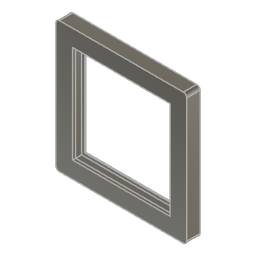
wand handle (Autodesk Fusion 360 archive; units mm, degrees)
design "noita spell v2"
Autodesk Fusion 360 part; units mm, degrees
sketch "Sketch1" plane through (0, 0, 0) normal (0, 1, 0) x (1, 0, 0)
  line L0 (0, 0) -> (38.1, 0)
  line L1 (38.1, 0) -> (38.1, -38.1)
  line L2 (38.1, -38.1) -> (0, -38.1)
  line L3 (0, -38.1) -> (0, 0)
  circle A0 centre (19.05, -40.55) radius 1.25
  line L4 (-4.9, -39.3) -> (43, -39.3) construction
  line L5 (-4.9, -41.8) -> (43, -41.8) construction
  line L6 (0, -19.05) -> (38.1, -19.05)
  line L7 (19.05, 0) -> (19.05, -38.1)
  line L8 (-3.65, 4.9) -> (41.75, 4.9)
  line L9 (43, 3.65) -> (43, -41.75)
  line L10 (41.75, -43) -> (-3.65, -43)
  line L11 (-4.9, -41.75) -> (-4.9, 3.65)
  circle A1 centre (-2.45, -40.55) radius 1.25
  line L12 (-3.7, -43) -> (-3.7, 4.9) construction
  line L13 (-1.2, -43) -> (-1.2, 4.9) construction
  line L14 (39.3, -43) -> (39.3, 4.9) construction
  line L15 (41.8, 4.9) -> (41.8, -43) construction
  line L16 (-4.9, 3.7) -> (43, 3.7) construction
  line L17 (43, 1.2) -> (-4.9, 1.2) construction
  circle A2 centre (40.55, -40.55) radius 1.25
  circle A3 centre (40.55, -19.05) radius 1.25
  circle A4 centre (40.55, 2.45) radius 1.25
  circle A5 centre (19.05, 2.45) radius 1.25
  circle A6 centre (-2.45, 2.45) radius 1.25
  circle A7 centre (-2.45, -19.05) radius 1.25
  arc A8 (-4.9, -41.75) -> (-3.65, -43) centre (-3.65, -41.75) ccw
  arc A9 (41.75, -43) -> (43, -41.75) centre (41.75, -41.75) ccw
  arc A10 (43, 3.65) -> (41.75, 4.9) centre (41.75, 3.65) ccw
  arc A11 (-3.65, 4.9) -> (-4.9, 3.65) centre (-3.65, 3.65) ccw
  line L18 (1.2, -36.9) -> (36.9, -36.9)
  line L19 (36.9, -36.9) -> (36.9, -1.2)
  line L20 (36.9, -1.2) -> (1.2, -1.2)
  line L21 (1.2, -1.2) -> (1.2, -36.9)
  dimension "d1" = 38.1
  dimension "d2" = 38.1
  dimension "d3" = 2.5
  dimension "d4" = 1.2
  dimension "d5" = 1.2
  dimension "d8" = 2.5
  dimension "d9" = 1.2
  dimension "d10" = 1.2
  dimension "d11" = 1.2
  dimension "d13" = 1.2
  dimension "d14" = 1.2
  dimension "d15" = 1.2
  dimension "d16" = 2.5
  dimension "d17" = 1.25
  dimension "d18" = 1.2
  dimension "d19" = 1.2
  dimension "d20" = 1.2
  dimension "d21" = 1.2
  constraint horizontal L0
  constraint vertical L1
  constraint horizontal L2
  constraint vertical L3
  constraint coincident L0.start L3.end
  constraint horizontal L4
  constraint tangent A0 L4
  constraint horizontal L5
  constraint tangent A0 L5
  constraint midpoint L3 L6.start
  constraint midpoint L1 L6.end
  constraint midpoint L0 L7.start
  constraint midpoint L2 L7.end
  constraint horizontal L8
  constraint vertical L9
  constraint horizontal L10
  constraint vertical L11
  constraint coincident L4.start L11
  constraint coincident L4.end L9
  constraint coincident L5.end L9
  constraint coincident L5.start L11
  constraint coincident A0.centre L7
  constraint coincident L10 L12.start
  constraint coincident L8 L12.end
  constraint perpendicular L8 L12
  constraint tangent A1 L12
  constraint coincident L10 L13.start
  constraint coincident L8 L13.end
  constraint perpendicular L8 L13
  constraint tangent A1 L13
  constraint coincident L10 L14.start
  constraint coincident L8 L14.end
  constraint perpendicular L8 L14
  constraint coincident L8 L15.start
  constraint coincident L10 L15.end
  constraint perpendicular L10 L15
  constraint coincident L11 L16.start
  constraint coincident L9 L16.end
  constraint perpendicular L9 L16
  constraint coincident L9 L17.start
  constraint coincident L11 L17.end
  constraint perpendicular L11 L17
  constraint tangent L4 A2
  constraint tangent L15 A2
  constraint tangent L14 A2
  constraint tangent L15 A3
  constraint tangent L16 A4
  constraint tangent L16 A5
  constraint tangent L12 A6
  constraint tangent L17 A6
  constraint tangent L16 A6
  constraint tangent L14 A4
  constraint tangent L15 A4
  constraint tangent L17 A5
  constraint tangent L17 A4
  constraint tangent L12 A7
  constraint tangent L13 A7
  constraint tangent L14 A3
  constraint coincident L6 A3.centre
  constraint coincident L6 A7.centre
  constraint coincident L7 A5.centre
  constraint tangent L5 A1
  constraint tangent L10 A8
  constraint tangent L11 A8
  constraint tangent L9 A9
  constraint tangent L10 A9
  constraint equal A8 A9
  constraint tangent L8 A10
  constraint tangent L9 A10
  constraint equal A8 A10
  constraint tangent L8 A11
  constraint tangent L11 A11
  constraint equal A8 A11
  constraint horizontal L18
  constraint vertical L19
  constraint horizontal L20
  constraint vertical L21
  measures "d1" distance of L1.end L2.end
  measures "d2" distance of L0.start L2.end
  measures "d3" diameter of A0
  measures "d4" distance of L2 L4
  measures "d5" distance of L5 L10
  measures "d8" diameter of A1
  measures "d9" distance of L11 L12
  measures "d10" distance of L3 L13
  measures "d11" distance of L1 L14
  measures "d13" distance of L9 L15
  measures "d14" distance of L8 L16
  measures "d15" distance of L0 L17
  measures "d16" diameter of A2
  measures "d17" radius of A8
  measures "d18" distance of L2 L18
  measures "d19" distance of L3 L21
  measures "d20" distance of L0 L20
  measures "d21" distance of L1 L19
extrude "Extrude1" add sketch "Sketch1" along normal blind 0.4 contours L0 L3 L6 L7 L20 L21 | L0 L1 L6 L7 L19 L20 | L2 L3 L6 L7 L18 L21 | L1 L2 L6 L7 L18 L19 | A0 | L8 L9 L10 L11 A8 A9 A10 A11 | A1 | A2 | A3 | A4 | A5 | A6 | A7
extrude "Extrude2" add sketch "Sketch1" against normal blind 4.1
ref_plane "WorkPlane1" through (19.05, -3.3782, 19.05) normal (0, -1, 0) x (-1, 0, 0)
sketch "Sketch2" plane through (0, -3.3782, 0) normal (0, -1, 0) x (-1, 0, 0)
  line L0 (-1.2, -1.2) -> (-1.2, -36.9)
  line L1 (-1.2, -36.9) -> (-36.9, -36.9)
  line L2 (-36.9, -36.9) -> (-36.9, -1.2)
  line L3 (-36.9, -1.2) -> (-1.2, -1.2)
  line L4 (0, -38.1) -> (0, 0)
  line L5 (0, 0) -> (-38.1, 0)
  line L6 (-38.1, 0) -> (-38.1, -38.1)
  line L7 (-38.1, -38.1) -> (0, -38.1)
extrude "Extrude3" add sketch "Sketch2" along normal up to surface (0.7218 mm away)
sketch "Sketch3" plane through (0, -4.1, 0) normal (0, -1, 0) x (1, 0, 0)
  line L0 (1.2, 36.9) -> (36.9, 36.9)
  line L1 (36.9, 36.9) -> (36.9, 1.2)
  line L2 (36.9, 1.2) -> (1.2, 1.2)
  line L3 (1.2, 1.2) -> (1.2, 36.9)
  circle A0 centre (40.55, 19.05) radius 1.25
  circle A1 centre (-2.45, 19.05) radius 1.25
  circle A2 centre (19.05, -2.45) radius 1.25
  circle A3 centre (40.55, 40.55) radius 1.25
  circle A4 centre (40.55, -2.45) radius 1.25
  circle A5 centre (19.05, 40.55) radius 1.25
  circle A6 centre (-2.45, -2.45) radius 1.25
  circle A7 centre (-2.45, 40.55) radius 1.25
  arc A8 (41.75, -4.9) -> (43, -3.65) centre (41.75, -3.65) ccw
  line L4 (43, -3.65) -> (43, 41.75)
  arc A9 (43, 41.75) -> (41.75, 43) centre (41.75, 41.75) ccw
  line L5 (41.75, 43) -> (-3.65, 43)
  arc A10 (-3.65, 43) -> (-4.9, 41.75) centre (-3.65, 41.75) ccw
  line L6 (-4.9, 41.75) -> (-4.9, -3.65)
  arc A11 (-4.9, -3.65) -> (-3.65, -4.9) centre (-3.65, -3.65) ccw
  line L7 (-3.65, -4.9) -> (41.75, -4.9)
extrude "Extrude4" add sketch "Sketch3" along normal blind 0.4 contours A0 | A1 | A2 | A3 | A4 | A5 | A6 | A7 | A8 L4 A9 L5 A10 L6 A11 L7
equation "d2 = d1"
equation "d5 = d4"
equation "d8 = d3"
equation "d9 = d5"
equation "d10 = d5"
equation "d11 = d5"
equation "d13 = d5"
equation "d14 = d5"
equation "d15 = d5"
equation "d16 = d3"
equation "d17 = d3 / 2"
equation "d19 = d18"
equation "d20 = d18"
equation "d21 = d18"
